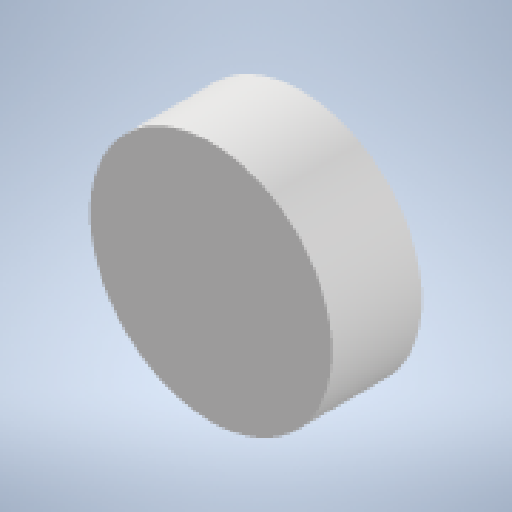
# Autodesk Inventor part: RightEyePeach
Saved by Autodesk Inventor 2023 (Build 270158000, 158)
## iProperties
Created: 2022-11-09
Part Number: RightEyePeach
Material: Generic
Document SubType Name: Modeling
Designer: reide
Density: 1 g/cm^3
Appearance: Default
Author: reide
Autodesk Inventor part; units mm, degrees
ref_plane "YZ Plane" through (0, 0, 0) normal (1, 0, 0) x (0, 1, 0)
ref_plane "XZ Plane" through (0, 0, 0) normal (0, 1, 0) x (-1, 0, 0)
ref_plane "XY Plane" through (0, 0, 0) normal (0, 0, 1) x (1, 0, 0)
sketch "Sketch1" plane through (0, 0, 0) normal (0, 0, 1) x (1, 0, 0)
  arc A0 (19.34, 27.5) -> (15.1432, 23.6188) centre (20.2446, 22.3122) ccw projected
  ellipse E0 centre (10.3798, 24.0498) end of major axis (5.6164, 24.4807) minor radius 4.1297 (15.017, 22.9479) -> (15.1432, 23.6188) ccw projected
  arc A1 (15.1432, 23.6188) -> (15.017, 22.9479) centre (20.2446, 22.3122) ccw projected
  ellipse E1 centre (10.3798, 24.0498) end of major axis (15.1432, 23.6188) minor radius 4.1297 (15.1432, 23.6188) -> (12.9076, 27.5) ccw projected
  line L0 (19.34, 27.5) -> (12.9076, 27.5) projected
  arc A2 (-39.3309, 27.5) -> (-40.6675, 25.4611) centre (-22.0465, 14.7112) ccw projected
  spline S0 degree 3 poles (-36.653, 23.7418) (-36.6606, 23.7128) (-36.6686, 23.684) (-36.7991, 23.2374) (-37.003, 22.8436) (-37.4852, 22.2335) (-37.7387, 21.9969) (-38.2828, 21.6418) (-38.5675, 21.5137) (-39.1231, 21.3843) (-39.3904, 21.368) (-39.8134, 21.4302) (-39.973, 21.4755) (-40.1234, 21.542) (-40.4076, 21.6676) (-40.656, 21.8705) (-40.9477, 22.2598) (-41.0339, 22.4145) (-41.2588, 22.9573) (-41.3118, 23.3772) (-41.242, 24.3141) (-41.0671, 24.8281) (-40.751, 25.3396) (-40.7103, 25.401) (-40.6675, 25.4611) knots -2.04297 -2.04297 -2.04297 -2.04297 -2.033998 -2.033998 -1.903383 -1.903383 -1.8007 -1.8007 -1.70847 -1.70847 -1.629539 -1.629539 -1.580207 -1.580207 -1.580207 -1.486994 -1.486994 -1.434286 -1.434286 -1.31073 -1.31073 -1.152429 -1.152429 -1.130329 -1.130329 -1.130329 -1.130329 projected
  arc A3 (-33.7904, 27.5) -> (-36.653, 23.7418) centre (-28.9143, 20.8166) ccw projected
  line L1 (-28.5459, 27.5) -> (-33.7904, 27.5) projected
  arc A4 (-28.5459, 27.5) -> (-24.1154, 23.7029) centre (-15.1131, 38.6898) ccw projected
  arc A5 (-24.1154, 23.7029) -> (-33.0724, 15.676) centre (-20.6959, 10.8762) ccw projected
  arc A6 (-33.0724, 15.676) -> (-34.9124, -1.3721) centre (-5.25, 4.0498) ccw projected
  arc A7 (-34.9124, -1.3721) -> (-41.9254, -12.6146) centre (-23.9, -16.0502) ccw projected
  arc A8 (-41.9254, -12.6146) -> (-28.5956, -16.8849) centre (-31, -1.4502) ccw projected
  arc A9 (-28.5956, -16.8849) -> (16.976, -25.5478) centre (-0.4792, 6.8253) ccw projected
  arc A10 (16.976, -25.5478) -> (30.0763, -26.2375) centre (24.3257, -10.7068) ccw projected
  arc A11 (30.0763, -26.2375) -> (27.2801, -16.1178) centre (15.4592, -24.8303) ccw projected
  arc A12 (27.2801, -16.1178) -> (29.9552, -2.5721) centre (8.0722, -5.2875) ccw projected
  arc A13 (29.9552, -2.5721) -> (23.4312, 19.4757) centre (20.2446, 6.5436) ccw projected
  arc A14 (23.4312, 19.4757) -> (21.0581, 26.5) centre (20.2446, 22.3122) ccw projected
  line L2 (21.0581, 26.5) -> (22.4374, 26.5) projected
  arc A15 (23.4374, 27.5) -> (22.4374, 26.5) centre (23.4374, 26.5) ccw projected
  line L3 (90.6006, 27.5) -> (23.4374, 27.5) projected
  line L4 (90.6006, 35.5016) -> (90.6006, 27.5) projected
  line L5 (-41.1756, 35.5016) -> (90.6006, 35.5016) projected
  arc A16 (-43.1756, 37.5016) -> (-41.1756, 35.5016) centre (-41.1756, 37.5016) ccw projected
  line L6 (-43.1756, 130.5) -> (-43.1756, 37.5016) projected
  arc A17 (-41.1756, 132.5) -> (-43.1756, 130.5) centre (-41.1756, 130.5) ccw projected
  line L7 (90.6006, 132.5) -> (-41.1756, 132.5) projected
  line L8 (90.6006, 140.5) -> (90.6006, 132.5) projected
  line L9 (-46.6006, 140.5) -> (90.6006, 140.5) projected
  arc A18 (-46.6006, 140.5) -> (-50.6006, 136.5) centre (-46.6006, 136.5) ccw projected
  line L10 (-50.6006, 31.5) -> (-50.6006, 136.5) projected
  arc A19 (-50.6006, 31.5) -> (-46.6006, 27.5) centre (-46.6006, 31.5) ccw projected
  line L11 (-39.3309, 27.5) -> (-46.6006, 27.5) projected
  ellipse E2 centre (9.5858, 24.0498) end of major axis (5.148, 24.0498) minor radius 3.9921 projected
  ellipse E3 centre (-7, 5) end of major axis (-10, 5) minor radius 2.4928 projected
  arc A20 (-34.1817, -3.1484) -> (-29.5706, -15.0085) centre (105.9158, 44.4945) ccw projected
  arc A21 (-39.7014, -11.76) -> (-29.5706, -15.0085) centre (-29.0305, 4.0974) ccw projected
  arc A22 (-34.1817, -3.1484) -> (-39.7014, -11.76) centre (-21.1644, -17.5666) ccw projected
  arc A23 (14.6041, 2.032) -> (13, 1) centre (14.3758, 0.6242) ccw projected
  arc A24 (13, 1) -> (11.0739, 2.9743) centre (10, 0) ccw projected
  ellipse E4 centre (12.8441, 3) end of major axis (12.8441, 12) minor radius 1.7702 (14.6041, 2.032) -> (11.0739, 2.9743) ccw projected
  circle A25 centre (22, -1.4502) radius 2.7388 projected
  circle A26 centre (0, 0) radius 2.8284 projected
  arc A27 (21.1775, -24.9987) -> (27.4696, -19.1953) centre (6.8467, -3.1484) ccw projected
  arc A28 (27.9278, -24.9172) -> (27.4696, -19.1953) centre (9.7342, -23.4947) ccw projected
  arc A29 (21.1775, -24.9987) -> (27.9278, -24.9172) centre (24.3663, -9.517) ccw projected
  ellipse E5 centre (20.2446, 22.5631) end of major axis (24.2633, 22.2872) minor radius 3.5714 projected
  ellipse E6 centre (28.4561, 1.7414) end of major axis (25.9246, 1.7414) minor radius 2.1289 projected
  circle A30 centre (0, 0) radius 2.687
  constraints: 1 centre point, 1 coincident, 6 other
extrude "Extrusion1" add sketch "Sketch1" along normal blind 2 contours A30
body "Solid1"
